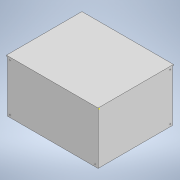
# Autodesk Inventor part: kevnat part2
Saved by Autodesk Inventor 2022 (Build 260153000, 153)
## iProperties
Created: 2023-03-07
Part Number: kevnat part2
Material: Generic
Document SubType Name: Modeling
Designer: Riordan
Density: 1 g/cm^3
Appearance: Default
Author: Riordan
Autodesk Inventor part; units mm, degrees
ref_plane "YZ Plane" through (0, 0, 0) normal (1, 0, 0) x (0, 1, 0)
ref_plane "XZ Plane" through (0, 0, 0) normal (0, 1, 0) x (-1, 0, 0)
ref_plane "XY Plane" through (0, 0, 0) normal (0, 0, 1) x (1, 0, 0)
sketch "Sketch1" plane through (0, 0, 0) normal (0, 1, 0) x (-1, 0, 0)
  line L0 (0, 0) -> (200, 0)
  line L1 (200, 0) -> (200, -150)
  line L2 (200, -150) -> (0, -150)
  line L3 (0, -150) -> (0, 0)
  dimension "d0" = 200
  dimension "d1" = 150
  constraints: 8 end point, 2 parallel, 1 horizontal, 1 perpendicular
  measures "d0" distance of L1.end L2.end
  measures "d1" distance of L0.end L1.end
extrude "Extrusion1" add sketch "Sketch1" along normal blind 2
sketch "Sketch2" plane through (0, 0, 0) normal (0, -1, 0) x (1, 0, 0)
  line L0 (-200, 0) -> (0, 0) projected
  line L1 (-200, 0) -> (-198, 0)
  line L2 (-198, 0) -> (-198, -2)
  line L3 (-198, -2) -> (-2, -2)
  line L4 (-2, -2) -> (-2, -148)
  line L5 (-2, -148) -> (0, -148)
  line L6 (0, 0) -> (0, -150) projected
  dimension "d4" = 2
  dimension "d5" = 2
  dimension "d6" = 196
  dimension "d7" = 146
  constraints: 10 end point, 4 perpendicular, 2 point on line
  measures "d4" distance of L0.start L1.end
  measures "d5" distance of L1.end L2.end
  measures "d6" distance of L2.end L3.end
  measures "d7" distance of L3.end L4.end
extrude "Extrusion2" add sketch "Sketch2" along normal blind 102
sketch "Sketch3" plane through (-200, 2, 0) normal (0, 0, 1) x (1, 0, 0)
  line L0 (0, -2) -> (2, -2) projected
  line L1 (2, -2) -> (6.5, -2)
  line L2 (198, -2) -> (2, -2) projected
  line L3 (6.5, -2) -> (6.5, -5.5)
  circle A0 centre (6.5, -5.5) radius 1
  line L4 (2, -104) -> (198, -104) projected
  line L5 (2, -104) -> (6.5, -104)
  line L6 (6.5, -104) -> (6.5, -99.5)
  circle A1 centre (6.5, -99.5) radius 1
  line L7 (200, -104) -> (2, -104) projected
  line L8 (200, -104) -> (194.5, -104)
  line L9 (194.5, -104) -> (194.5, -99.5)
  circle A2 centre (194.5, -99.5) radius 1
  point P0 (200, -2)
  dimension "d10" = 4.5
  dimension "d11" = 3.5
  dimension "d12" = 2
  dimension "d13" = 4.5
  dimension "d14" = 4.5
  dimension "d15" = 5.5
  constraints: 12 end point, 3 centre point, 3 coincident, 3 point on line, 2 perpendicular, 1 vertical
  measures "d10" distance of L0.end L1.end
  measures "d11" distance of L1.end L3.end
  measures "d12" diameter of A0
  measures "d13" distance of L4.start L5.end
  measures "d14" distance of L5.end L6.end
  measures "d15" distance of L7.start L8.end
extrude "Extrusion3" cut sketch "Sketch3" against normal blind 10
sketch "Sketch4" plane through (0, 2, 0) normal (1, 0, 0) x (0, 0, -1)
  line L0 (148, -2) -> (148, -104) projected
  line L1 (148, -2) -> (143.5, -2)
  line L2 (150, -2) -> (0, -2) projected
  line L3 (143.5, -2) -> (143.5, -5.5)
  line L4 (148, -104) -> (143.5, -104)
  line L5 (143.5, -104) -> (143.5, -99.5)
  line L6 (143.5, -99.5) -> (148, -99.5)
  line L7 (148, -99.5) -> (148, -104)
  circle A0 centre (143.5, -99.5) radius 1
  circle A1 centre (143.5, -5.5) radius 1
  dimension "d18" = 4.5
  dimension "d19" = 3.5
  dimension "d20" = 4.5
  dimension "d21" = 4.5
  dimension "d22" = 2
  constraints: 12 end point, 2 centre point, 2 coincident, 2 parallel, 2 perpendicular, 1 horizontal, 1 point on line
  measures "d18" distance of L0.start L1.end
  measures "d19" distance of L1.end L3.end
  measures "d20" distance of L5.end L6.end
  measures "d21" distance of L4.end L5.end
  measures "d22" diameter of A0
extrude "Extrusion4" cut sketch "Sketch4" against normal blind 10 contours A1 | A0 L5 L6 | L6 L5 A0
sketch "Sketch5" plane through (0, 0, 0) normal (0, -1, 0) x (1, 0, 0)
  line L0 (-2, -148) -> (-2, -2) projected
  line L1 (-2, -75) -> (-172, -75)
  line L2 (-200, -150) -> (-200, 0) projected
  line L3 (-172, -75) -> (-174, -75)
  line L4 (-172, -75) -> (-172, -2)
  line L5 (-2, -2) -> (-198, -2) projected
  line L6 (0, -150) -> (-200, -150) projected
  line L7 (-172, -2) -> (-2, -2)
  line L8 (-2, -2) -> (-2, -150)
  line L9 (-2, -150) -> (-172, -150)
  line L10 (-172, -150) -> (-172, -2)
  line L11 (-200, 0) -> (0, 0) projected
  line L12 (-174, 0) -> (-2, 0)
  line L13 (-2, 0) -> (-2, -150)
  line L14 (-2, -150) -> (-174, -150)
  line L15 (-174, -150) -> (-174, 0)
  dimension "d28" = 170
  dimension "d29" = 2
  constraints: 22 end point, 4 parallel, 4 point on line, 3 horizontal, 3 perpendicular, 1 midpoint, 1 vertical
  measures "d28" distance of L1.start L1.end
  measures "d29" distance of L1.end L3.end
sketch "Sketch6" plane through (-2, 0, -2) normal (0, 0, -1) x (-1, 0, 0)
  point P0 (-2, 0)
extrude "Extrusion5" cut sketch "Sketch5" along normal mid plane 1000 contours L15 L6 L2 L11
sketch "Sketch7" plane through (0, 0, 0) normal (0, -1, 0) x (1, 0, 0)
  line L0 (-174, -2) -> (-2, -2) projected
  line L1 (-174, -2) -> (-172, -2)
  line L2 (-172, -2) -> (-172, 0)
  line L3 (-174, 0) -> (0, 0) projected
  line L4 (-174, 0) -> (-172, 0)
  line L5 (-174, 0) -> (-174, -2)
  dimension "d32" = 2
  constraints: 8 end point, 2 perpendicular, 2 point on line, 1 collinear
  measures "d32" distance of L0.start L1.end
extrude "Extrusion6" cut sketch "Sketch7" along normal blind 1000
sketch "Sketch9" plane through (0, 0, 0) normal (0, -1, 0) x (1, 0, 0)
  line L0 (0, -148) -> (0, 0) projected
  line L1 (0, -74) -> (-182, -74)
  line L2 (-174, 0) -> (-174, -150) projected
  line L3 (-174, 0) -> (-182, 0)
  line L4 (-182, 0) -> (-182, -150)
  line L5 (-182, -150) -> (-174, -150)
  line L6 (-174, -150) -> (-174, 0)
  dimension "d44" = 182
  constraints: 10 end point, 2 horizontal, 2 parallel, 1 midpoint, 1 perpendicular
  measures "d44" distance of L1.start L1.end
extrude "Extrusion8" add sketch "Sketch9" against normal blind 2
sketch "Sketch10" plane through (-2, -102, -2) normal (0, 0, -1) x (-1, 0, 0)
  line L0 (180, 102) -> (-2, 102) projected
  line L1 (180, 102) -> (178, 102)
  line L2 (170, 102) -> (170, 0) projected
  line L3 (178, 102) -> (170, 102)
  line L4 (170, 102) -> (170, 0)
  line L5 (170, 0) -> (178, 0)
  line L6 (178, 0) -> (178, 102)
  dimension "d47" = 2
  constraints: 10 end point, 2 parallel, 1 horizontal, 1 perpendicular, 1 point on line
  measures "d47" distance of L0.start L1.end
extrude "Extrusion9" add sketch "Sketch10" against normal blind 2
sketch "Sketch11" plane through (-2, -102, -2) normal (0, 0, -1) x (-1, 0, 0)
  line L0 (0, 102) -> (178, 102) projected
  line L1 (178, 102) -> (178, 98.5)
  line L2 (178, 0) -> (178, 102) projected
  line L3 (178, 98.5) -> (173.5, 98.5)
  line L4 (178, 0) -> (0, 0) projected
  line L5 (178, 0) -> (173.5, 0)
  line L6 (173.5, 0) -> (173.5, 4.5)
  circle A0 centre (173.5, 98.5) radius 1
  circle A1 centre (173.5, 4.5) radius 1
  point P0 (-2, 102)
  dimension "d50" = 3.5
  dimension "d51" = 4.5
  dimension "d52" = 4.5
  dimension "d53" = 2
  constraints: 8 end point, 2 centre point, 2 coincident, 2 perpendicular, 2 point on line
  measures "d50" distance of L0.end L1.end
  measures "d51" distance of L1.end L3.end
  measures "d52" distance of L5.end L6.end
  measures "d53" diameter of A0
extrude "Extrusion10" cut sketch "Sketch11" against normal blind 2
body "Solid1"
